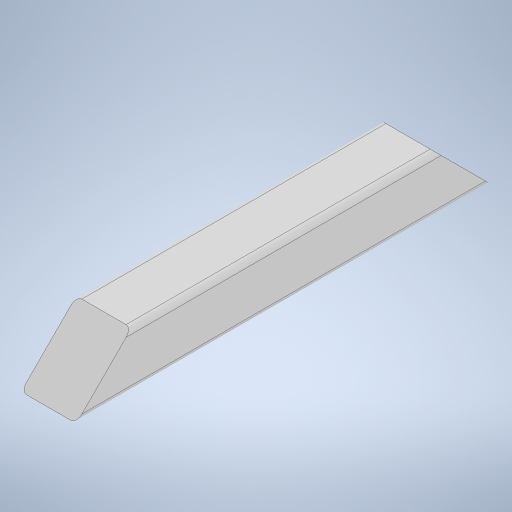
# Autodesk Inventor part: item40x40_1000
Saved by Autodesk Inventor 2024.4 (Build 284460000, 460)
## iProperties
Created: 2025-11-05
Part Number: item40x40_1000
Material: Generic
Document SubType Name: Modeling
Designer: jonas
Density: 1 g/cm^3
Appearance: Default
Author: jonas
Autodesk Inventor part; units mm, degrees
ref_plane "YZ Plane" through (0, 0, 0) normal (1, 0, 0) x (0, 1, 0)
ref_plane "XZ Plane" through (0, 0, 0) normal (0, 1, 0) x (-1, 0, 0)
ref_plane "XY Plane" through (0, 0, 0) normal (0, 0, 1) x (1, 0, 0)
sketch "Sketch1" plane through (0, 0, 0) normal (0, 1, 0) x (-1, 0, 0)
  line L0 (0, 12.4728) -> (0, -12.4728) construction
  line L1 (2.135, 0) -> (-2.135, 0) construction
  line L2 (16, 20) -> (-16, 20)
  line L3 (-20, 16) -> (-20, -16)
  line L4 (-16, -20) -> (16, -20)
  line L5 (20, -16) -> (20, 16)
  arc A0 (-16, 20) -> (-20, 16) centre (-16, 16) ccw
  arc A1 (-20, -16) -> (-16, -20) centre (-16, -16) ccw
  arc A2 (16, -20) -> (20, -16) centre (16, -16) ccw
  arc A3 (20, 16) -> (16, 20) centre (16, 16) ccw
  point P0 (0, 0)
  point P1 (0, 0)
  dimension "d1" = 4
  dimension "d2" = 4
  dimension "d3" = 40
  constraints: 12 end point, 8 point on circle, 8 tangent, 4 centre point, 2 equal radius, 2 horizontal, 2 midpoint, 2 parallel, 2 perpendicular, 1 coincident, 1 vertical, 2 other
  measures "d1" radius of A0
  measures "d2" radius of A2
  measures "d3" distance between parallel lines of L2 L4
extrude "Extrusion1" add sketch "Sketch1" along normal blind 300
sketch "Sketch2" plane through (20, 0, 16) normal (1, 0, 0) x (0, 0, -1)
  line L0 (36, 0) -> (-4, 40)
  line L1 (-4, 40) -> (-4, 0)
  line L2 (-4, 0) -> (36, 0)
  line L3 (-4, 300) -> (-4, 260)
  line L4 (-4, 260) -> (36, 300)
  line L5 (36, 300) -> (-4, 300)
  line L6 (-4, 0) -> (-4, 300) projected
  line L7 (36, 0) -> (36, 300) projected
  point P0 (16, 0)
  dimension "d6" = 45
  dimension "d7" = 45
  constraints: 12 end point, 3 point on line, 2 perpendicular, 1 vertical
  measures "d6" angle of L0 L1
  measures "d7" angle of L4 L3
extrude "Extrusion2" cut sketch "Sketch2" against normal through all contours L2 L1 L0 | L4 L3 L5
body "Solid1"
